axle_mount (Autodesk Fusion 360 design; units mm, degrees)
Autodesk Fusion 360 part; units mm, degrees
sketch "Sketch1" plane through (0, 0, 0) normal (0, 1, 0) x (1, 0, 0)
  circle A0 centre (0, 0) radius 15
  circle A1 centre (0, 0) radius 4.5
  line L0 (-12, 9) -> (12, 9)
  line L1 (-12, 9) -> (-25, 9)
  line L2 (-25, 9) -> (-25, -5)
  line L3 (-25, -5) -> (25, -5)
  line L4 (25, -5) -> (25, 9)
  line L5 (25, 9) -> (12, 9)
  dimension "d1" = 9
  dimension "d2" = 30
  dimension "d3" = 9
  dimension "d6" = 25
  dimension "d7" = 25
  dimension "d8" = 14
  constraint coincident A0.centre A1.centre
  constraint coincident A0 L0.start
  constraint coincident A0 L0.end
  constraint horizontal L0
  constraint parallel L0 L1
  constraint perpendicular L1 L2
  constraint perpendicular L2 L3
  constraint perpendicular L3 L4
  constraint perpendicular L4 L5
  measures "d1" diameter of A1
  measures "d2" diameter of A0
  measures "d3" distance of A0.centre L0
  measures "d6" distance of A0.centre L2
  measures "d7" distance of A0.centre L4
  measures "d8" distance of L3 L5
extrude "Extrude1" add sketch "Sketch1" along normal blind 50 contours A0 L0 L3 | A0 L3 L4 L5 | A0 L3 | A0 L1 L2 L3
sketch "Sketch2" plane through (0, 0, -9) normal (0, 0, -1) x (1, 0, 0)
  line L0 (25, 0) -> (-25, 0)
  line L1 (-25, 0) -> (-25, -50)
  line L2 (-25, -50) -> (25, -50)
  line L3 (25, -50) -> (25, 0)
  line L4 (0, 0) -> (0, -50)
  circle A0 centre (-15, -12) radius 3.5
  circle A1 centre (-15, -37) radius 3.5
  circle A2 centre (15, -12) radius 3.5
  circle A3 centre (15, -37) radius 3.5
  dimension "d9" = 15
  dimension "d10" = 15
  dimension "d11" = 25
  dimension "d12" = 12
  dimension "d13" = 7
  dimension "d14" = 7
  constraint coincident L4.start origin
  constraint midpoint L2 L4.end
  constraint symmetric L4 A0 A2
  constraint symmetric L4 A1 A3
  measures "d9" distance of L4 A0.centre
  measures "d10" distance of L4 A1.centre
  measures "d11" distance of A0.centre A1.centre
  measures "d12" distance of L0 A0.centre
  measures "d13" diameter of A0
  measures "d14" diameter of A1
sketch "Sketch3" plane through (0, 50, 0) normal (0, 1, 0) x (-1, 0, 0)
  circle A0 centre (0, 0) radius 4.5
  line L0 (-25, -9) -> (25, -9)
  line L1 (25, -9) -> (25, 5)
  line L2 (25, 5) -> (14.1421, 5)
  arc A1 (14.1421, 5) -> (-14.1421, 5) centre (0, 0) ccw
  line L3 (-14.1421, 5) -> (-25, 5)
  line L4 (-25, 5) -> (-25, -9)
  circle A2 centre (0, 0) radius 9.5
  dimension "d15" = 19
  constraint concentric A0 A2
  measures "d15" diameter of A2
sketch "Sketch4" plane through (0, 0, 5) normal (0, 0, 1) x (-1, 0, 0)
  line L0 (-14.1421, -50) -> (-14.1421, 0)
  line L1 (-14.1421, 0) -> (-25, 0)
  line L2 (-25, 0) -> (-25, -50)
  line L3 (-25, -50) -> (-14.1421, -50)
  line L4 (0, 0) -> (0, -41)
  line L5 (-14.1421, -15) -> (-25, -15)
  line L6 (-25, -15) -> (-25, 0)
  line L7 (-25, 0) -> (-14.1421, 0)
  line L8 (-14.1421, 0) -> (-14.1421, -15)
  line L9 (14.1421, -15) -> (25, -15)
  line L10 (14.1421, 0) -> (14.1421, -15)
  line L11 (25, 0) -> (14.1421, 0)
  line L12 (25, -15) -> (25, 0)
  dimension "d20" = 15
  constraint coincident L4.start origin
  constraint vertical L4
  constraint horizontal L5
  constraint vertical L6
  constraint horizontal L7
  constraint vertical L8
  constraint coincident L2 L1.end
  constraint symmetric L4 L5.start L9.start
  constraint symmetric L4 L5.end L9.end
  constraint symmetric L4 L1.end L11.start
  constraint symmetric L4 L0.end L10.start
  constraint collinear L1 L7
  measures "d20" distance of L5.end L1.end
extrude "Extrude3" cut sketch "Sketch2" against normal blind 26 contours A0 | A1 | A2 | A3
extrude "Extrude2" cut sketch "Sketch3" against normal blind 23 contours L0 A2 picked at (-0.1121, -7.4958)
extrude "Extrude4" [suppressed]
equation "d7 = d6"
equation "d10 = d9"
equation "d14 = d13"
